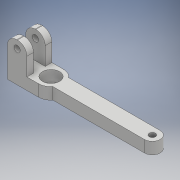
# Autodesk Inventor part: tiller rotation bracket
Saved by Autodesk Inventor 2017 (Build 210142000, 142)
## iProperties
Created: 2017-12-08
Part Number: tiller rotation bracket
Material: Generic
Document SubType Name: Modeling
Designer: RLanting
Density: 1 g/cm^3
Appearance: Default
Author: RLanting
Autodesk Inventor part; units mm, degrees
ref_plane "YZ Plane" through (0, 0, 0) normal (1, 0, 0) x (0, 1, 0)
ref_plane "XZ Plane" through (0, 0, 0) normal (0, 1, 0) x (-1, 0, 0)
ref_plane "XY Plane" through (0, 0, 0) normal (0, 0, 1) x (1, 0, 0)
sketch "Sketch1" plane through (0, 0, 0) normal (0, 0, 1) x (1, 0, 0)
  line L0 (0, 0) -> (-40, 0) construction
  line L1 (0, 16) -> (-40, 16)
  line L2 (-40, -16) -> (0, -16)
  arc A0 (0, -16) -> (0, 16) centre (0, 0) ccw
  arc A1 (-40, 16) -> (-40, -16) centre (-40, 0) ccw construction
  circle A2 centre (0, 0) radius 11
  line L3 (-40, 16) -> (-40, -16)
  point P0 (-20, 0)
  dimension "d0" = 22
  dimension "d1" = 5
  dimension "d2" = 40
  constraints: 10 end point, 4 point on circle, 4 tangent, 3 centre point, 1 coincident, 1 horizontal, 1 midpoint, 1 parallel, 1 vertical
  measures "d0" diameter of A2
  measures "d1" radial gap between concentric circles of A0 A2
  measures "d2" distance of L0.start L0.end
extrude "Extrusion1" add sketch "Sketch1" along normal blind 15
sketch "Sketch2" plane through (0, 0, 15) normal (0, 0, 1) x (1, 0, 0)
  line L0 (0, 16) -> (-40, 16) projected
  line L1 (-40, 16) -> (-15, 16)
  line L2 (-15, 16) -> (-15, 7.5)
  line L3 (-15, 7.5) -> (-40, 7.5)
  line L4 (-40, 7.5) -> (-40, 16)
  line L5 (-40, 16) -> (-40, -16) projected
  line L6 (-40, -16) -> (-15, -16)
  line L7 (-15, -16) -> (-15, -7.5)
  line L8 (-15, -7.5) -> (-40, -7.5)
  line L9 (-40, -7.5) -> (-40, -16)
  point P0 (0, 0)
  dimension "d5" = 25
  dimension "d6" = 15
  constraints: 16 end point, 4 parallel, 2 horizontal, 2 perpendicular, 1 collinear, 1 point on line
  measures "d5" distance of L2.end L3.end
  measures "d6" distance between parallel lines of L8 L3
extrude "Extrusion2" add sketch "Sketch2" along normal blind 35
sketch "Sketch3" plane through (-40, -16, 0) normal (0, -1, 0) x (1, 0, 0)
  line L0 (0, 15) -> (25, 15) projected
  line L1 (0, 50) -> (25, 50) construction
  line L2 (12.5, 50) -> (12.5, 40) construction
  circle A0 centre (12.5, 40) radius 4
  point P0 (40, 0)
  dimension "d9" = 8
  dimension "d10" = 10
  constraints: 2 end point, 1 centre point, 1 coincident, 1 midpoint, 1 vertical
  measures "d9" diameter of A0
  measures "d10" distance of L2.start L2.end
extrude "Extrusion3" cut sketch "Sketch3" against normal through all
fillet "Fillet1" radius 12 4 edges at (-15, 11.75, 50) (-40, 11.75, 50) (-15, -11.75, 50) (-40, -11.75, 50)
sketch "Sketch4" plane through (0, 0, 0) normal (0, 0, -1) x (-1, 0, 0)
  circle A0 centre (0, 0) radius 11 projected
  circle A1 centre (0, 0) radius 8
  dimension "d14" = 16
  constraints: 1 centre point, 1 coincident
  measures "d14" diameter of A1
extrude "Extrusion4" add sketch "Sketch4" against normal blind 1
sketch "Sketch5" plane through (0, 0, 0) normal (0, 0, -1) x (-1, 0, 0)
  arc A0 (-120, 50) -> (-120, -50) centre (0, 0) ccw construction
  line L0 (0, 0) -> (-120, 50) construction
  circle A1 centre (0, 0) radius 11 construction
  line L1 (0, 0) -> (-120, -50) construction
  line L2 (0, 0) -> (-130, 0) construction
  line L3 (-120, 50) -> (-120, -50) construction
  line L4 (0, 0) -> (-130, 0) construction
  line L5 (0, 10) -> (-12.49, 10)
  line L6 (-130, -10) -> (-12.49, -10)
  arc A2 (0, -10) -> (0, 10) centre (0, 0) ccw
  arc A3 (-130, 10) -> (-130, -10) centre (-130, 0) ccw
  circle A4 centre (-130, 0) radius 4
  arc A5 (0, 16) -> (0, -16) centre (0, 0) ccw projected
  arc A6 (-12.49, 10) -> (-12.49, -10) centre (0, 0) ccw
  line L7 (-12.49, 10) -> (-130, 10)
  line L8 (-12.49, -10) -> (0, -10)
  point P0 (-65, 0)
  dimension "d17" = 100
  dimension "d18" = 130
  dimension "d19" = 45.24
  dimension "d20" = 10
  dimension "d21" = 8
  constraints: 20 end point, 10 point on circle, 8 tangent, 5 centre point, 4 parallel, 3 coincident, 1 collinear, 1 horizontal, 1 midpoint, 1 vertical
  measures "d17" distance of L0.end L1.end
  measures "d18" distance of L1.start L2.end
  measures "d19" angle of L1 L0
  measures "d20" radius of A2
  measures "d21" diameter of A4
extrude "Extrusion5" add sketch "Sketch5" against normal up to surface (15 mm away) contours A5 L6 A3 L7
body "Solid1"
